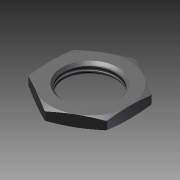
# Autodesk Inventor part: AT526
Saved by Autodesk Inventor 2011 SP1 (Build 150282100, 282)
## iProperties
Created: 2016-09-01
Part Number: AT526
Catalog Web Link: www.cadenas.de
Description: AT526 - Hex Mounting Nut-
Vendor: NKKSWITCHES
Document SubType Name: Modeling
Designer: psAdmin
Manufacturer: NKKSWITCHES
Mass: 0.199579 g
Surface Area: 3.39547 cm^2
Volume: 0.199579 cm^3
Density: 1 g/cm^3
Category: PARTsolutions
Company: NKKSWITCHES
Title: AT526
Author: Cadenas PARTsolutions
PSOL_IDENT_0: {$CADENAS_DATA\23d-libs\nkkswitches\rotary\hs_12_amp\parts\at526.prj},170 {VTYP=3D},{NB=AT526},{LINA=
PSOL_IDENT_1: AT526},{NN=AT526 - Hex Mounting Nut},{DATE=22.09.2015 06:04:15},{GEOMDATE=27.03.2009 08:52:00},{VERS
PSOL_IDENT_2: ION=},{LINEID=10},{LINESUBID=-1},{WBVAR=}  {NB=AT526},{LINA=AT526},{KT=DUMMY},{PN=AT526},{ND=10},{PI
PSOL_IDENT_3: TCH=0.75}
NN: AT526 - Hex Mounting Nut
NB: AT526
NBSYN: $PN.
LINA: AT526
PN: AT526
SUPPLIER: NKKSWITCHES
ARTICLENO: AT526
BOMINFO: AT526
CREATOR: CADENAS GmbH
Autodesk Inventor part; units mm, degrees
sketch "Sketch_1" plane through (0, 0, 0) normal (0, 0, 1) x (1, 0, 0)
  line L0 (0, -1.0033) -> (0, 1.0033)
  line L1 (4.594, 0.5973) -> (4.594, -0.5973)
  line L2 (4.594, -0.5973) -> (5, -1.0033)
  line L3 (5, -1.0033) -> (6.9977, -1.0033)
  line L4 (6.9977, -1.0033) -> (8.001, -0.7345)
  line L5 (8.001, -0.7345) -> (8.001, 0.7345)
  line L6 (8.001, 0.7345) -> (6.9977, 1.0033)
  line L7 (6.9977, 1.0033) -> (5, 1.0033)
  line L8 (5, 1.0033) -> (4.594, 0.5973)
  constraints: 18 end point
revolve "Revolution1" add sketch "Sketch_1" angle 360 about axis through (0, -1.0033, 0) along (0, -1, 0)
thread "Thread1" size "M10x0.75" class "6H" standard "ISO Metric profile" full length
sketch "Sketch_2" plane through (0, 0, 0) normal (0, 1, 0) x (-1, 0, 0)
  line L0 (13.9954, 8.0802) -> (0, 16.1605)
  line L1 (0, 16.1605) -> (-13.9954, 8.0802)
  line L2 (-13.9954, 8.0802) -> (-13.9954, -8.0802)
  line L3 (-13.9954, -8.0802) -> (0, -16.1605)
  line L4 (0, -16.1605) -> (13.9954, -8.0802)
  line L5 (13.9954, -8.0802) -> (13.9954, 8.0802)
  line L6 (6.9977, 4.0401) -> (0, 8.0802)
  line L7 (0, 8.0802) -> (-6.9977, 4.0401)
  line L8 (-6.9977, 4.0401) -> (-6.9977, -4.0401)
  line L9 (-6.9977, -4.0401) -> (0, -8.0802)
  line L10 (0, -8.0802) -> (6.9977, -4.0401)
  line L11 (6.9977, -4.0401) -> (6.9977, 4.0401)
  constraints: 24 end point
extrude "Extrusion1" cut sketch "Sketch_2" along normal mid plane 4.0132
ref_plane "1_XY" through (0, 0, 0) normal (0, 1, 0) x (1, 0, 0)
ref_plane "1_YZ" through (0, 0, 0) normal (1, 0, 0) x (0, 0, -1)
ref_plane "1_ZX" through (0, 0, 0) normal (0, 0, -1) x (0, 1, 0)
body "Solid1"
